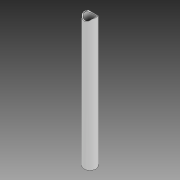
# Autodesk Inventor part: FE-110-002 Upright Middle Section
Saved by Autodesk Inventor 2021 (Build 250183000, 183)
## iProperties
Created: 2021-01-11
Part Number: FE-110-002 Upright Middle Section
Material: Aluminum 6061
Document SubType Name: Modeling
Density: 2.7 g/cm^3
Appearance: Aluminum - Dark
Autodesk Inventor part; units mm, degrees
ref_plane "YZ Plane" through (0, 0, 0) normal (1, 0, 0) x (0, 1, 0)
ref_plane "XZ Plane" through (0, 0, 0) normal (0, 1, 0) x (-1, 0, 0)
ref_plane "XY Plane" through (0, 0, 0) normal (0, 0, 1) x (1, 0, 0)
sketch "Sketch1" plane through (0, 0, 0) normal (0, 1, 0) x (-1, 0, 0)
  circle A0 centre (0, 0) radius 21.082
  circle A1 centre (0, 0) radius 17.526
  dimension "d0" = 42.164
  dimension "d1" = 35.052
  constraints: 2 centre point, 2 coincident
  measures "d0" diameter of A0
  measures "d1" diameter of A1
extrude "Extrusion1" add sketch "Sketch1" along normal mid plane 469.1126
sketch "Sketch2" plane through (0, 0, 0) normal (0, 0, 1) x (1, 0, 0)
  circle A0 centre (0, 245.7006) radius 21.082
  line L0 (21.082, 234.5563) -> (-21.082, 234.5563) projected
  line L1 (-21.082, -234.5563) -> (21.082, -234.5563) projected
  line L2 (-21.082, -234.5563) -> (-21.082, 234.5563) projected
  arc A1 (-21.082, -231.3813) -> (-17.907, -234.5563) centre (-17.907, -231.3813) ccw
  point P0 (0, 0)
  dimension "d4" = 42.164
  dimension "d6" = 11.1442
  dimension "d7" = 6.35
  constraints: 2 centre point, 2 point on circle, 2 point on line, 2 tangent, 1 vertical alignment
  measures "d4" diameter of A0
  measures "d6" distance from line of A0.centre L0
  measures "d7" diameter of A1
extrude "Extrusion2" cut sketch "Sketch2" against normal through all both and the other way through all
body "Solid1"
